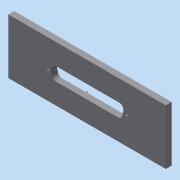
# Autodesk Inventor part: dsub37_cutout
Saved by Autodesk Inventor 2016 (Build 200138000, 138)
## iProperties
Created: 2016-10-18
Part Number: dsub37_cutout
Material: Generic
Document SubType Name: Modeling
Designer: Zara
Density: 1 g/cm^3
Appearance: Default
Author: Zara
Autodesk Inventor part; units mm, degrees
ref_plane "YZ Plane" through (0, 0, 0) normal (1, 0, 0) x (0, 1, 0)
ref_plane "XZ Plane" through (0, 0, 0) normal (0, 1, 0) x (-1, 0, 0)
ref_plane "XY Plane" through (0, 0, 0) normal (0, 0, 1) x (1, 0, 0)
sketch "Sketch1" plane through (0, 0, 0) normal (0, 0, 1) x (1, 0, 0)
  line L0 (-63.5, -22.225) -> (63.5, -22.225)
  line L1 (63.5, -22.225) -> (63.5, 22.225)
  line L2 (63.5, 22.225) -> (-63.5, 22.225)
  line L3 (-63.5, 22.225) -> (-63.5, -22.225)
  line L4 (-63.5, -22.225) -> (63.5, 22.225) construction
  line L5 (63.5, -22.225) -> (-63.5, 22.225) construction
  point P0 (0, 0)
  dimension "d0" = 127
  dimension "d1" = 44.45
  constraints: 12 end point, 2 midpoint, 2 parallel, 1 horizontal, 1 perpendicular
  measures "d0" distance of L1.end L2.end
  measures "d1" distance of L0.end L1.end
extrude "Extrusion1" add sketch "Sketch1" along normal blind 4.7498
sketch "Sketch2" plane through (0, 0, 4.7498) normal (0, 0, 1) x (1, 0, 0)
  point P0 (0, 0)
sketch "Sketch3" plane through (0, 0, 4.7498) normal (0, 0, 1) x (1, 0, 0)
  line L0 (-63.5, -22.225) -> (63.5, -22.225) construction
  line L1 (63.5, -22.225) -> (63.5, 22.225) construction
  line L2 (63.5, 22.225) -> (-63.5, 22.225) construction
  line L3 (-63.5, 22.225) -> (-63.5, -22.225) construction
  line L4 (0, 22.225) -> (0, -22.225) construction
  circle A0 centre (-31.75, 0) radius 1.1303
  circle A1 centre (31.75, 0) radius 1.1303
  line L5 (-31.75, 0) -> (31.75, 0) construction
  line L6 (-26.0604, 5.334) -> (26.0604, 5.334)
  line L7 (-24.9301, -5.461) -> (24.9301, -5.461)
  arc A2 (29.292, 1.088) -> (26.0604, 5.334) centre (26.0604, 1.9812) ccw
  arc A3 (24.9301, -5.461) -> (28.1617, -3.0014) centre (24.9301, -2.1082) ccw
  arc A4 (-26.0604, 5.334) -> (-29.292, 1.088) centre (-26.0604, 1.9812) ccw
  line L8 (-29.292, 1.088) -> (-28.1617, -3.0014)
  line L9 (29.292, 1.088) -> (28.1617, -3.0014)
  arc A5 (-28.1617, -3.0014) -> (-24.9301, -5.461) centre (-24.9301, -2.1082) ccw
  line L10 (29.292, 1.088) -> (29.292, -4.9317) construction
  point P0 (0, 0)
  point P1 (0, 5.334)
  point P2 (0, -5.461)
  point P3 (-28.9913, 0)
  point P4 (-30.6197, 0)
  point P5 (-28.9913, 0)
  point P6 (-30.6197, 0)
  point P7 (-30.6197, 0)
  point P8 (-28.9913, 0)
  point P9 (28.9913, 0)
  dimension "d7" = 2.2606
  dimension "d8" = 2.2606
  dimension "d9" = 63.5
  dimension "d11" = 6.7056
  dimension "d13" = 6.7056
  dimension "d15" = 52.1208
  dimension "d16" = 49.8602
  dimension "d17" = 10.795
  dimension "d20" = 5.334
  dimension "d24" = 3.3528
  dimension "d25" = 3.3528
  constraints: 14 end point, 8 point on circle, 8 tangent, 7 point on line, 6 midpoint, 5 centre point, 5 coincident, 3 horizontal, 1 horizontal alignment, 1 vertical, 2 other
  measures "d8" diameter of A1
  measures "d9" distance of L5.end L5.start
  measures "d11" diameter of A2
  measures "d13" diameter of A4
  measures "d15" distance of A2.centre A4.centre
  measures "d16" distance of A3.centre A5.centre
  measures "d17" distance between parallel lines of L6 L7
  measures "d20" distance from line of L6 L5.start
  measures "d24" radius of A3
  measures "d25" radius of A5
extrude "Extrusion2" cut sketch "Sketch3" against normal blind 4.7498
body "Solid1"
